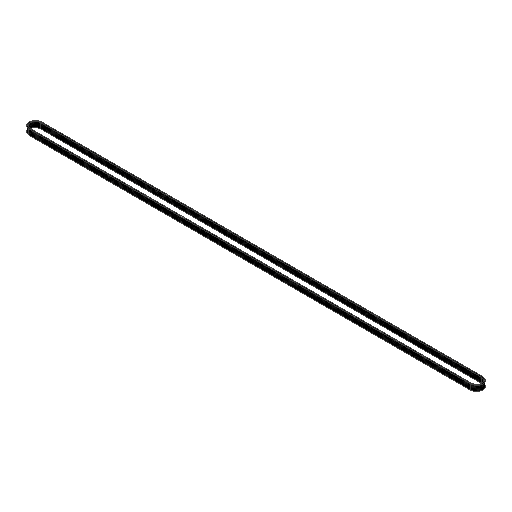
# Autodesk Inventor part: COTS_GENERIC_Y_Axis_Timing_Belt
Saved by Autodesk Inventor 2026.1 (Build 301233000, 233)
## iProperties
Created: 2017-05-25
Part Number: COTS_GENERIC_Y_Axis_Timing_Belt
Material: Ogólny
Document SubType Name: Modeling
Designer: Andrzej
Density: 1 g/cm^3
Appearance: Czarny
Mass: 9.5441 g
Surface Area: 166.643 cm^2
Volume: 9.5441 cm^3
Author: Andrzej
Autodesk Inventor part; units mm, degrees
ref_plane "YZ Plane" through (0, 0, 0) normal (1, 0, 0) x (0, 1, 0)
ref_plane "XZ Plane" through (0, 0, 0) normal (0, 1, 0) x (-1, 0, 0)
ref_plane "XY Plane" through (0, 0, 0) normal (0, 0, 1) x (1, 0, 0)
sketch "Szkic1" plane through (0, 0, 0) normal (0, 0, 1) x (1, 0, 0)
  line L0 (260, 0) -> (-260, 0) construction
  line L1 (260, 6) -> (-260, 6)
  line L2 (-260, -6) -> (260, -6)
  arc A0 (260, -6) -> (260, 6) centre (260, 0) ccw
  arc A1 (-260, 6) -> (-260, -6) centre (-260, 0) ccw
  line L3 (-260, 7.4) -> (260, 7.4)
  arc A2 (260, -7.4) -> (260, 7.4) centre (260, 0) ccw
  line L4 (260, -7.4) -> (-260, -7.4)
  arc A3 (-260, 7.4) -> (-260, -7.4) centre (-260, 0) ccw
  point P0 (0, 0)
  dimension "d0" = 260
  dimension "d1" = 12
  dimension "d2" = 1.4
  constraints: 12 end point, 8 point on circle, 4 centre point, 4 tangent, 2 parallel, 1 horizontal, 1 midpoint, 3 other
  measures "d0" distance of point (0, 0) L0.end
  measures "d1" diameter of A1
  measures "d2" distance between parallel lines of L1 L3
extrude "Wyciągnięcie proste1" add sketch "Szkic1" along normal blind 6.3
